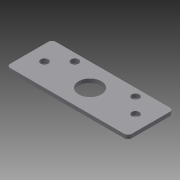
# Autodesk Inventor part: motorMount
Saved by Autodesk Inventor 2013 (Build 170138000, 138)
## iProperties
Created: 2012-12-12
Part Number: motorMount
Material: Generic
Document SubType Name: Modeling
Designer: istvan.burbank
Density: 1 g/cm^3
Author: istvan.burbank
Autodesk Inventor part; units mm, degrees
ref_plane "YZ Plane" through (0, 0, 0) normal (1, 0, 0) x (0, 1, 0)
ref_plane "XZ Plane" through (0, 0, 0) normal (0, 1, 0) x (-1, 0, 0)
ref_plane "XY Plane" through (0, 0, 0) normal (0, 0, 1) x (1, 0, 0)
sketch "Sketch1" plane through (0, 0, 0) normal (0, 1, 0) x (-1, 0, 0)
  line L0 (3.175, 0) -> (98.425, 0)
  line L1 (101.6, 3.175) -> (101.6, 34.925)
  line L2 (98.425, 38.1) -> (3.175, 38.1)
  line L3 (0, 34.925) -> (0, 3.175)
  arc A0 (3.175, 38.1) -> (0, 34.925) centre (3.175, 34.925) ccw
  arc A1 (101.6, 34.925) -> (98.425, 38.1) centre (98.425, 34.925) ccw
  arc A2 (98.425, 0) -> (101.6, 3.175) centre (98.425, 3.175) ccw
  arc A3 (0, 3.175) -> (3.175, 0) centre (3.175, 3.175) ccw
  point P0 (0, 0)
  point P1 (101.6, 38.1)
  point P2 (101.6, 0)
  point P3 (0, 38.1)
  dimension "d0" = 101.6
  dimension "d1" = 38.1
  dimension "d13" = 3.175
  constraints: 8 end point, 8 point on circle, 8 point on line, 8 tangent, 4 centre point, 3 equal radius, 2 parallel, 1 horizontal, 1 perpendicular
  measures "d0" distance of point (0, 38.1) point (101.6, 38.1)
  measures "d1" distance of point (101.6, 38.1) point (101.6, 0)
  measures "d13" radius of A0
extrude "Extrusion1" add sketch "Sketch1" along normal blind 3.175
sketch "Sketch2" plane through (0, 3.175, 0) normal (0, 1, 0) x (1, 0, 0)
  line L0 (-3.175, 0) -> (-98.425, 0) projected
  line L1 (-101.6, -3.175) -> (-101.6, -34.925) projected
  line L2 (0, -34.925) -> (0, -3.175) projected
  point P0 (0, 0)
  point P1 (-76.2, 0)
  point P2 (-76.2, -76.2)
  point P3 (-50.8, -19.05)
  dimension "d4" = 50.8
  dimension "d5" = 19.05
  dimension "d29" = 50.8
  constraints: 1 other
  measures "d5" distance from line of L0 point (-50.8, -19.05)
  measures "d29" distance from line of L2 point (-50.8, -19.05)
hole "Hole1" at (-50.8, 3.175, 19.05) direction (0, -1, 0) diameter 19.05 end through all
sketch "Sketch3" plane through (0, 3.175, 0) normal (0, 1, 0) x (1, 0, 0)
  line L0 (0, -34.925) -> (0, -3.175) projected
  line L1 (-101.6, -3.175) -> (-101.6, -34.925) projected
  circle A0 centre (-50.8, -19.05) radius 9.525 projected
  point P0 (0, 0)
  point P1 (-76.2, -6.35)
  point P2 (-25.4, -6.35)
  point P3 (-12.7, -19.05)
  point P4 (-88.9, -19.05)
  dimension "d19" = 50.8
  dimension "d20" = 25.4
  dimension "d21" = 25.4
  dimension "d30" = 12.7
  dimension "d31" = 12.7
  dimension "d33" = 12.7
  constraints: 3 horizontal alignment
  measures "d19" distance of point (-25.4, -6.35) point (-76.2, -6.35)
  measures "d20" distance from line of L1 point (-76.2, -6.35)
  measures "d21" distance from line of L0 point (-25.4, -6.35)
  measures "d30" horizontal distance of point (-12.7, -19.05) point (-25.4, -6.35)
  measures "d31" horizontal distance of point (-88.9, -19.05) point (-76.2, -6.35)
  measures "d33" horizontal distance of point (-12.7, -19.05) point (-25.4, -6.35)
hole "Hole2" at (-76.2, 3.175, 6.35) at (-25.4, 3.175, 6.35) at (-12.7, 3.175, 19.05) at (-88.9, 3.175, 19.05) direction (0, -1, 0) diameter 6.35 end through all
equation "\"d4\" = d29"
equation "\"d20\" = d21"
body "Solid1"
